Autodesk Inventor part; units mm, degrees
(part 2 of 2)
sketch "Sketch3" plane through (0, 0, 6) normal (0, 0, 1) x (1, 0, 0)
  spline S0 degree 3 poles (20.5297, 43.2466) (22.2295, 43.4705) (23.9405, 43.387) (25.6486, 43.3844) (26.304, 43.3834) (26.9616, 43.2869) (27.6139, 43.2016) (28.7287, 43.056) (29.8441, 42.908) (30.9514, 42.7157) (31.5862, 42.6054) (32.2139, 42.4329) (32.8297, 42.2404) (33.8935, 41.9078) (34.9839, 41.623) (35.9513, 41.0534) (36.6965, 40.6147) (37.4233, 40.1316) (38.101, 39.5959) (38.7184, 39.1078) (39.283, 38.5455) (39.8274, 37.9745) (40.65, 37.1119) (41.2721, 36.1125) (41.7344, 35.009) (41.9858, 34.409) (42.2171, 33.807) (42.3148, 33.1626) (42.3838, 32.7068) (42.4311, 32.2477) (42.4863, 31.7898) (42.5051, 31.6342) (42.5379, 31.4772) (42.5307, 31.3223) (42.5103, 30.883) (42.4889, 30.4426) (42.4376, 30.0063) (42.3757, 29.4795) (42.3242, 28.9459) (42.1926, 28.4346) (42.0204, 27.7655) (41.7834, 27.1124) (41.5557, 26.4588) (41.4533, 26.1649) (41.2846, 25.8939) (41.1845, 25.5995) (41.0297, 25.1443) (40.6487, 24.9481) (40.2751, 24.735) (39.0786, 24.0524) (37.7888, 23.6132) (36.4604, 23.2756) (36.4092, 23.2626) (36.3519, 23.2739) (36.2541, 23.2739) (36.4505, 24.0942) (36.6431, 24.8992) (36.8482, 25.7561) (36.6342, 25.7121) (36.4556, 25.6842) (36.2819, 25.6384) (34.8048, 25.2487) (33.3458, 24.8006) (31.9384, 24.2032) (30.8391, 23.7366) (29.7481, 23.2495) (28.6622, 22.7525) (27.9303, 22.4174) (27.21, 22.0565) (26.4914, 21.6935) (25.9143, 21.4019) (25.3477, 21.0895) (24.7091, 20.7508) (24.8093, 21.0975) (24.9023, 21.38) (24.9722, 21.6681) (25.2788, 22.9311) (25.5986, 24.1916) (25.8741, 25.4615) (26.054, 26.2911) (26.177, 27.1338) (26.3051, 27.9737) (26.3899, 28.5302) (26.4541, 29.091) (26.4995, 29.6521) (26.5622, 30.4281) (26.6152, 31.2056) (26.6412, 31.9834) (26.6645, 32.6834) (26.6815, 33.387) (26.6382, 34.0851) (26.5457, 35.5779) (26.2672, 37.0419) (25.7848, 38.4586) (25.5349, 39.1927) (25.1548, 39.8693) (24.7123, 40.5097) (23.7382, 41.9194) (22.4265, 42.8309) (20.7539, 43.2161) (20.6807, 43.2329) (20.6045, 43.2367) (20.5297, 43.2466) knots 0 0 0 0 1 1 1 2 2 2 3 3 3 4 4 4 5 5 5 6 6 6 7 7 7 8 8 8 9 9 9 10 10 10 11 11 11 12 12 12 13 13 13 14 14 14 15 15 15 16 16 16 17 17 17 18 18 18 19 19 19 20 20 20 21 21 21 22 22 22 23 23 23 24 24 24 25 25 25 26 26 26 27 27 27 28 28 28 29 29 29 30 30 30 31 31 31 32 32 32 33 33 33 34 34 34 34
  line L0 (20.5297, 43.2466) -> (22.2295, 43.4705) construction
  line L1 (22.2295, 43.4705) -> (23.9405, 43.387) construction
  line L2 (23.9405, 43.387) -> (25.6486, 43.3844) construction
  line L3 (25.6486, 43.3844) -> (26.304, 43.3834) construction
  line L4 (26.304, 43.3834) -> (26.9616, 43.2869) construction
  line L5 (26.9616, 43.2869) -> (27.6139, 43.2016) construction
  line L6 (27.6139, 43.2016) -> (28.7287, 43.056) construction
  line L7 (28.7287, 43.056) -> (29.8441, 42.908) construction
  line L8 (29.8441, 42.908) -> (30.9514, 42.7157) construction
  line L9 (30.9514, 42.7157) -> (31.5862, 42.6054) construction
  line L10 (31.5862, 42.6054) -> (32.2139, 42.4329) construction
  line L11 (32.2139, 42.4329) -> (32.8297, 42.2404) construction
  line L12 (32.8297, 42.2404) -> (33.8935, 41.9078) construction
  line L13 (33.8935, 41.9078) -> (34.9839, 41.623) construction
  line L14 (34.9839, 41.623) -> (35.9513, 41.0534) construction
  line L15 (35.9513, 41.0534) -> (36.6965, 40.6147) construction
  line L16 (36.6965, 40.6147) -> (37.4233, 40.1316) construction
  line L17 (37.4233, 40.1316) -> (38.101, 39.5959) construction
  line L18 (38.101, 39.5959) -> (38.7184, 39.1078) construction
  line L19 (38.7184, 39.1078) -> (39.283, 38.5455) construction
  line L20 (39.283, 38.5455) -> (39.8274, 37.9745) construction
  line L21 (39.8274, 37.9745) -> (40.65, 37.1119) construction
  line L22 (40.65, 37.1119) -> (41.2721, 36.1125) construction
  line L23 (41.2721, 36.1125) -> (41.7344, 35.009) construction
  line L24 (41.7344, 35.009) -> (41.9858, 34.409) construction
  line L25 (41.9858, 34.409) -> (42.2171, 33.807) construction
  line L26 (42.2171, 33.807) -> (42.3148, 33.1626) construction
  line L27 (42.3148, 33.1626) -> (42.3838, 32.7068) construction
  line L28 (42.3838, 32.7068) -> (42.4311, 32.2477) construction
  line L29 (42.4311, 32.2477) -> (42.4863, 31.7898) construction
  line L30 (42.4863, 31.7898) -> (42.5051, 31.6342) construction
  line L31 (42.5051, 31.6342) -> (42.5379, 31.4772) construction
  line L32 (42.5379, 31.4772) -> (42.5307, 31.3223) construction
  line L33 (42.5307, 31.3223) -> (42.5103, 30.883) construction
  line L34 (42.5103, 30.883) -> (42.4889, 30.4426) construction
  line L35 (42.4889, 30.4426) -> (42.4376, 30.0063) construction
  line L36 (42.4376, 30.0063) -> (42.3757, 29.4795) construction
  line L37 (42.3757, 29.4795) -> (42.3242, 28.9459) construction
  line L38 (42.3242, 28.9459) -> (42.1926, 28.4346) construction
  line L39 (42.1926, 28.4346) -> (42.0204, 27.7655) construction
  line L40 (42.0204, 27.7655) -> (41.7834, 27.1124) construction
  line L41 (41.7834, 27.1124) -> (41.5557, 26.4588) construction
  line L42 (41.5557, 26.4588) -> (41.4533, 26.1649) construction
  line L43 (41.4533, 26.1649) -> (41.2846, 25.8939) construction
  line L44 (41.2846, 25.8939) -> (41.1845, 25.5995) construction
  line L45 (41.1845, 25.5995) -> (41.0297, 25.1443) construction
  line L46 (41.0297, 25.1443) -> (40.6487, 24.9481) construction
  line L47 (40.6487, 24.9481) -> (40.2751, 24.735) construction
  line L48 (40.2751, 24.735) -> (39.0786, 24.0524) construction
  line L49 (39.0786, 24.0524) -> (37.7888, 23.6132) construction
  line L50 (37.7888, 23.6132) -> (36.4604, 23.2756) construction
  line L51 (36.4604, 23.2756) -> (36.4092, 23.2626) construction
  line L52 (36.4092, 23.2626) -> (36.3519, 23.2739) construction
  line L53 (36.3519, 23.2739) -> (36.2541, 23.2739) construction
  line L54 (36.2541, 23.2739) -> (36.4505, 24.0942) construction
  line L55 (36.4505, 24.0942) -> (36.6431, 24.8992) construction
  line L56 (36.6431, 24.8992) -> (36.8482, 25.7561) construction
  line L57 (36.8482, 25.7561) -> (36.6342, 25.7121) construction
  line L58 (36.6342, 25.7121) -> (36.4556, 25.6842) construction
  line L59 (36.4556, 25.6842) -> (36.2819, 25.6384) construction
  line L60 (36.2819, 25.6384) -> (34.8048, 25.2487) construction
  line L61 (34.8048, 25.2487) -> (33.3458, 24.8006) construction
  line L62 (33.3458, 24.8006) -> (31.9384, 24.2032) construction
  line L63 (31.9384, 24.2032) -> (30.8391, 23.7366) construction
  line L64 (30.8391, 23.7366) -> (29.7481, 23.2495) construction
  line L65 (29.7481, 23.2495) -> (28.6622, 22.7525) construction
  line L66 (28.6622, 22.7525) -> (27.9303, 22.4174) construction
  line L67 (27.9303, 22.4174) -> (27.21, 22.0565) construction
  line L68 (27.21, 22.0565) -> (26.4914, 21.6935) construction
  line L69 (26.4914, 21.6935) -> (25.9143, 21.4019) construction
  line L70 (25.9143, 21.4019) -> (25.3477, 21.0895) construction
  line L71 (25.3477, 21.0895) -> (24.7091, 20.7508) construction
  line L72 (24.7091, 20.7508) -> (24.8093, 21.0975) construction
  line L73 (24.8093, 21.0975) -> (24.9023, 21.38) construction
  line L74 (24.9023, 21.38) -> (24.9722, 21.6681) construction
  line L75 (24.9722, 21.6681) -> (25.2788, 22.9311) construction
  line L76 (25.2788, 22.9311) -> (25.5986, 24.1916) construction
  line L77 (25.5986, 24.1916) -> (25.8741, 25.4615) construction
  line L78 (25.8741, 25.4615) -> (26.054, 26.2911) construction
  line L79 (26.054, 26.2911) -> (26.177, 27.1338) construction
  line L80 (26.177, 27.1338) -> (26.3051, 27.9737) construction
  line L81 (26.3051, 27.9737) -> (26.3899, 28.5302) construction
  line L82 (26.3899, 28.5302) -> (26.4541, 29.091) construction
  line L83 (26.4541, 29.091) -> (26.4995, 29.6521) construction
  line L84 (26.4995, 29.6521) -> (26.5622, 30.4281) construction
  line L85 (26.5622, 30.4281) -> (26.6152, 31.2056) construction
  line L86 (26.6152, 31.2056) -> (26.6412, 31.9834) construction
  line L87 (26.6412, 31.9834) -> (26.6645, 32.6834) construction
  line L88 (26.6645, 32.6834) -> (26.6815, 33.387) construction
  line L89 (26.6815, 33.387) -> (26.6382, 34.0851) construction
  line L90 (26.6382, 34.0851) -> (26.5457, 35.5779) construction
  line L91 (26.5457, 35.5779) -> (26.2672, 37.0419) construction
  line L92 (26.2672, 37.0419) -> (25.7848, 38.4586) construction
  line L93 (25.7848, 38.4586) -> (25.5349, 39.1927) construction
  line L94 (25.5349, 39.1927) -> (25.1548, 39.8693) construction
  line L95 (25.1548, 39.8693) -> (24.7123, 40.5097) construction
  line L96 (24.7123, 40.5097) -> (23.7382, 41.9194) construction
  line L97 (23.7382, 41.9194) -> (22.4265, 42.8309) construction
  line L98 (22.4265, 42.8309) -> (20.7539, 43.2161) construction
  line L99 (20.7539, 43.2161) -> (20.6807, 43.2329) construction
  line L100 (20.6807, 43.2329) -> (20.6045, 43.2367) construction
  line L101 (20.6045, 43.2367) -> (20.5297, 43.2466) construction
  spline S1 degree 3 poles (36.6036, 23.5895) (37.0569, 23.702) (37.5183, 23.7768) (37.9504, 23.9327) (38.6597, 24.1886) (39.3668, 24.4661) (39.9357, 24.9927) (40.1802, 25.219) (40.2083, 25.5928) (39.8107, 25.7537) (39.4496, 25.8997) (39.0786, 25.933) (38.6918, 25.8914) (38.254, 25.8443) (37.8103, 25.844) (37.3764, 25.7764) (37.2463, 25.7562) (37.07, 25.5981) (37.0357, 25.4707) (36.8712, 24.8601) (36.7483, 24.2385) (36.6036, 23.5895) knots 0 0 0 0 1 1 1 2 2 2 3 3 3 4 4 4 5 5 5 6 6 6 7 7 7 7
  line L102 (36.6036, 23.5895) -> (37.0569, 23.702) construction
  line L103 (37.0569, 23.702) -> (37.5183, 23.7768) construction
  line L104 (37.5183, 23.7768) -> (37.9504, 23.9327) construction
  line L105 (37.9504, 23.9327) -> (38.6597, 24.1886) construction
  line L106 (38.6597, 24.1886) -> (39.3668, 24.4661) construction
  line L107 (39.3668, 24.4661) -> (39.9357, 24.9927) construction
  line L108 (39.9357, 24.9927) -> (40.1802, 25.219) construction
  line L109 (40.1802, 25.219) -> (40.2083, 25.5928) construction
  line L110 (40.2083, 25.5928) -> (39.8107, 25.7537) construction
  line L111 (39.8107, 25.7537) -> (39.4496, 25.8997) construction
  line L112 (39.4496, 25.8997) -> (39.0786, 25.933) construction
  line L113 (39.0786, 25.933) -> (38.6918, 25.8914) construction
  line L114 (38.6918, 25.8914) -> (38.254, 25.8443) construction
  line L115 (38.254, 25.8443) -> (37.8103, 25.844) construction
  line L116 (37.8103, 25.844) -> (37.3764, 25.7764) construction
  line L117 (37.3764, 25.7764) -> (37.2463, 25.7562) construction
  line L118 (37.2463, 25.7562) -> (37.07, 25.5981) construction
  line L119 (37.07, 25.5981) -> (37.0357, 25.4707) construction
  line L120 (37.0357, 25.4707) -> (36.8712, 24.8601) construction
  line L121 (36.8712, 24.8601) -> (36.7483, 24.2385) construction
  line L122 (36.7483, 24.2385) -> (36.6036, 23.5895) construction
  line L123 (20.3717, 33.3225) -> (30.5343, 33.3225) construction
  line L124 (30.5343, 33.3225) -> (30.5343, 28.6993) construction
  line L125 (30.5343, 28.6993) -> (20.3717, 28.6993) construction
  line L126 (20.3717, 28.6993) -> (20.3717, 33.3225) construction
  spline S2 degree 2 poles (21.5765, 30.0395) (21.2323, 30.0395) (20.7494, 30.1833) (20.5361, 30.2861) knots 0 0 0 1 2 2 2
  line L127 (20.5361, 30.2861) -> (20.5361, 30.8153)
  line L128 (20.5361, 30.8153) -> (20.567, 30.8153)
  spline S3 degree 2 poles (20.567, 30.8153) (20.7751, 30.62) (21.3017, 30.4043) (21.5457, 30.4043) knots 0 0 0 1 2 2 2
  spline S4 degree 2 poles (21.5457, 30.4043) (21.8951, 30.4043) (22.2522, 30.6945) (22.2522, 30.9334) knots 0 0 0 1 2 2 2
  spline S5 degree 2 poles (22.2522, 30.9334) (22.2522, 31.1235) (22.0646, 31.3599) (21.8617, 31.419) knots 0 0 0 1 2 2 2
  spline S6 degree 2 poles (21.8617, 31.419) (21.7153, 31.4601) (21.4712, 31.5166) (21.2888, 31.5628) knots 0 0 0 1 2 2 2
  spline S7 degree 2 poles (21.2888, 31.5628) (21.1244, 31.6065) (20.865, 31.7375) (20.7648, 31.8428) knots 0 0 0 1 2 2 2
  spline S8 degree 2 poles (20.7648, 31.8428) (20.6672, 31.9482) (20.5593, 32.2307) (20.5593, 32.4157) knots 0 0 0 1 2 2 2
  spline S9 degree 2 poles (20.5593, 32.4157) (20.5593, 32.801) (21.1604, 33.3225) (21.6254, 33.3225) knots 0 0 0 1 2 2 2
  spline S10 degree 2 poles (21.6254, 33.3225) (21.8925, 33.3225) (22.3652, 33.2172) (22.5681, 33.117) knots 0 0 0 1 2 2 2
  line L129 (22.5681, 33.117) -> (22.5681, 32.6135)
  line L130 (22.5681, 32.6135) -> (22.5373, 32.6135)
  spline S11 degree 2 poles (22.5373, 32.6135) (22.3857, 32.7522) (21.9131, 32.9577) (21.6536, 32.9577) knots 0 0 0 1 2 2 2
  spline S12 degree 2 poles (21.6536, 32.9577) (21.3608, 32.9577) (20.9985, 32.6829) (20.9985, 32.4594) knots 0 0 0 1 2 2 2
  spline S13 degree 2 poles (20.9985, 32.4594) (20.9985, 32.259) (21.2118, 32.0201) (21.4121, 31.9661) knots 0 0 0 1 2 2 2
  spline S14 degree 2 poles (21.4121, 31.9661) (21.5457, 31.9302) (21.9336, 31.8377) (22.0621, 31.7992) knots 0 0 0 1 2 2 2
  spline S15 degree 2 poles (22.0621, 31.7992) (22.3883, 31.699) (22.6914, 31.2957) (22.6914, 31.0002) knots 0 0 0 1 2 2 2
  spline S16 degree 2 poles (22.6914, 31.0002) (22.6914, 30.8127) (22.5399, 30.4531) (22.4037, 30.3272) knots 0 0 0 1 2 2 2
  spline S17 degree 2 poles (22.4037, 30.3272) (22.2522, 30.1885) (21.8668, 30.0395) (21.5765, 30.0395) knots 0 0 0 1 2 2 2
  spline S18 degree 2 poles (25.0831, 31.3496) (25.0831, 30.7536) (24.5153, 30.0497) (24.0812, 30.0497) knots 0 0 0 1 2 2 2
  spline S19 degree 2 poles (24.0812, 30.0497) (23.904, 30.0497) (23.6316, 30.132) (23.4904, 30.2167) knots 0 0 0 1 2 2 2
  line L131 (23.4904, 30.2167) -> (23.4904, 29.22)
  line L132 (23.4904, 29.22) -> (23.0896, 29.22)
  line L133 (23.0896, 29.22) -> (23.0896, 32.4748)
  line L134 (23.0896, 32.4748) -> (23.4904, 32.4748)
  line L135 (23.4904, 32.4748) -> (23.4904, 32.2256)
  spline S20 degree 2 poles (23.4904, 32.2256) (23.6394, 32.3617) (24.0041, 32.5416) (24.2174, 32.5416) knots 0 0 0 1 2 2 2
  spline S21 degree 2 poles (24.2174, 32.5416) (24.6258, 32.5416) (25.0831, 31.8942) (25.0831, 31.3496) knots 0 0 0 1 2 2 2
  spline S22 degree 2 poles (24.6695, 31.3034) (24.6695, 31.7118) (24.41, 32.1614) (24.1197, 32.1614) knots 0 0 0 1 2 2 2
  spline S23 degree 2 poles (24.1197, 32.1614) (23.9502, 32.1614) (23.6316, 32.0098) (23.4904, 31.8916) knots 0 0 0 1 2 2 2
  line L136 (23.4904, 31.8916) -> (23.4904, 30.5404)
  spline S24 degree 2 poles (23.4904, 30.5404) (23.6471, 30.4659) (23.8706, 30.4094) (24.0144, 30.4094) knots 0 0 0 1 2 2 2
  spline S25 degree 2 poles (24.0144, 30.4094) (24.3252, 30.4094) (24.6695, 30.8667) (24.6695, 31.3034) knots 0 0 0 1 2 2 2
  line L137 (25.9077, 30.096) -> (25.5069, 30.096)
  line L138 (25.5069, 30.096) -> (25.5069, 32.4748)
  line L139 (25.5069, 32.4748) -> (25.9077, 32.4748)
  line L140 (25.9077, 32.4748) -> (25.9077, 30.096)
  line L141 (25.9359, 32.8704) -> (25.4812, 32.8704)
  line L142 (25.4812, 32.8704) -> (25.4812, 33.2865)
  line L143 (25.4812, 33.2865) -> (25.9359, 33.2865)
  line L144 (25.9359, 33.2865) -> (25.9359, 32.8704)
  point P0 (-33.7147, -35.2257)
  point P1 (-33.0448, -40.4532)
  point P2 (-33.7217, -38.9912)
  point P3 (-33.1276, -39.7943)
  point P4 (-39.3868, -42.9109)
  point P5 (0, 0)
  constraints: 5 other
extrude "Extrusion4" cut sketch "Sketch3" against normal blind 0.5
sketch "Sketch4" plane through (0, 0, 6) normal (0, 0, 1) x (1, 0, 0)
  line L0 (26.9346, 33.3438) -> (41.0814, 33.3438) construction
  line L1 (41.0814, 33.3438) -> (41.0814, 29.9657) construction
  line L2 (41.0814, 29.9657) -> (26.9346, 29.9657) construction
  line L3 (26.9346, 29.9657) -> (26.9346, 33.3438) construction
  line L4 (29.524, 30.0325) -> (29.0513, 30.0325)
  line L5 (29.0513, 30.0325) -> (27.6487, 32.7658)
  line L6 (27.6487, 32.7658) -> (27.6487, 30.0325)
  line L7 (27.6487, 30.0325) -> (27.2557, 30.0325)
  line L8 (27.2557, 30.0325) -> (27.2557, 33.2025)
  line L9 (27.2557, 33.2025) -> (27.8542, 33.2025)
  line L10 (27.8542, 33.2025) -> (29.131, 30.6927)
  line L11 (29.131, 30.6927) -> (29.131, 33.2025)
  line L12 (29.131, 33.2025) -> (29.524, 33.2025)
  line L13 (29.524, 33.2025) -> (29.524, 30.0325)
  line L14 (32.4346, 30.0325) -> (31.9619, 30.0325)
  line L15 (31.9619, 30.0325) -> (30.5593, 32.7658)
  line L16 (30.5593, 32.7658) -> (30.5593, 30.0325)
  line L17 (30.5593, 30.0325) -> (30.1662, 30.0325)
  line L18 (30.1662, 30.0325) -> (30.1662, 33.2025)
  line L19 (30.1662, 33.2025) -> (30.7648, 33.2025)
  line L20 (30.7648, 33.2025) -> (32.0415, 30.6927)
  line L21 (32.0415, 30.6927) -> (32.0415, 33.2025)
  line L22 (32.0415, 33.2025) -> (32.4346, 33.2025)
  line L23 (32.4346, 33.2025) -> (32.4346, 30.0325)
  spline S0 degree 2 poles (34.3715, 30.2843) (34.3227, 30.2483) (34.1583, 30.1199) (34.0812, 30.0813) knots 0 0 0 1 2 2 2
  spline S1 degree 2 poles (34.0812, 30.0813) (33.9759, 30.0248) (33.7781, 29.9657) (33.5983, 29.9657) knots 0 0 0 1 2 2 2
  spline S2 degree 2 poles (33.5983, 29.9657) (33.4518, 29.9657) (33.1872, 30.0762) (33.0871, 30.1764) knots 0 0 0 1 2 2 2
  spline S3 degree 2 poles (33.0871, 30.1764) (32.992, 30.274) (32.8764, 30.5617) (32.8764, 30.721) knots 0 0 0 1 2 2 2
  spline S4 degree 2 poles (32.8764, 30.721) (32.8764, 30.9676) (33.0845, 31.317) (33.3105, 31.4171) knots 0 0 0 1 2 2 2
  spline S5 degree 2 poles (33.3105, 31.4171) (33.5109, 31.5096) (34.0555, 31.579) (34.3715, 31.597) knots 0 0 0 1 2 2 2
  line L24 (34.3715, 31.597) -> (34.3715, 31.674)
  spline S6 degree 2 poles (34.3715, 31.674) (34.3715, 31.8128) (34.2867, 31.9849) (34.2097, 32.0337) knots 0 0 0 1 2 2 2
  spline S7 degree 2 poles (34.2097, 32.0337) (34.1326, 32.0825) (33.9117, 32.1133) (33.7935, 32.1133) knots 0 0 0 1 2 2 2
  spline S8 degree 2 poles (33.7935, 32.1133) (33.6548, 32.1133) (33.2797, 32.0311) (33.0922, 31.9515) knots 0 0 0 1 2 2 2
  line L25 (33.0922, 31.9515) -> (33.0691, 31.9515)
  line L26 (33.0691, 31.9515) -> (33.0691, 32.3599)
  spline S9 degree 2 poles (33.0691, 32.3599) (33.1795, 32.3908) (33.5931, 32.4678) (33.7961, 32.4678) knots 0 0 0 1 2 2 2
  spline S10 degree 2 poles (33.7961, 32.4678) (34.0427, 32.4678) (34.3792, 32.3908) (34.5128, 32.2906) knots 0 0 0 1 2 2 2
  spline S11 degree 2 poles (34.5128, 32.2906) (34.6438, 32.193) (34.7722, 31.8821) (34.7722, 31.6586) knots 0 0 0 1 2 2 2
  line L27 (34.7722, 31.6586) -> (34.7722, 30.0325)
  line L28 (34.7722, 30.0325) -> (34.3715, 30.0325)
  line L29 (34.3715, 30.0325) -> (34.3715, 30.2843)
  line L30 (34.3715, 30.6182) -> (34.3715, 31.2784)
  spline S12 degree 2 poles (34.3715, 31.2784) (34.2276, 31.2656) (33.7935, 31.2219) (33.6573, 31.1808) knots 0 0 0 1 2 2 2
  spline S13 degree 2 poles (33.6573, 31.1808) (33.4981, 31.132) (33.29, 30.9291) (33.29, 30.7492) knots 0 0 0 1 2 2 2
  spline S14 degree 2 poles (33.29, 30.7492) (33.29, 30.5437) (33.5212, 30.3357) (33.7421, 30.3357) knots 0 0 0 1 2 2 2
  spline S15 degree 2 poles (33.7421, 30.3357) (33.9296, 30.3357) (34.2379, 30.4975) (34.3715, 30.6182) knots 0 0 0 1 2 2 2
  line L31 (37.3052, 30.0325) -> (36.7785, 30.0325)
  line L32 (36.7785, 30.0325) -> (35.8948, 31.1808)
  line L33 (35.8948, 31.1808) -> (35.7356, 31.0267)
  line L34 (35.7356, 31.0267) -> (35.7356, 30.0325)
  line L35 (35.7356, 30.0325) -> (35.3348, 30.0325)
  line L36 (35.3348, 30.0325) -> (35.3348, 33.3438)
  line L37 (35.3348, 33.3438) -> (35.7356, 33.3438)
  line L38 (35.7356, 33.3438) -> (35.7356, 31.4069)
  line L39 (35.7356, 31.4069) -> (36.6758, 32.4113)
  line L40 (36.6758, 32.4113) -> (37.1741, 32.4113)
  line L41 (37.1741, 32.4113) -> (36.198, 31.4171)
  line L42 (36.198, 31.4171) -> (37.3052, 30.0325)
  spline S16 degree 2 poles (38.5382, 29.9786) (37.9679, 29.9786) (37.3411, 30.6182) (37.3411, 31.2091) knots 0 0 0 1 2 2 2
  spline S17 degree 2 poles (37.3411, 31.2091) (37.3411, 31.7896) (37.9499, 32.4781) (38.4406, 32.4781) knots 0 0 0 1 2 2 2
  spline S18 degree 2 poles (38.4406, 32.4781) (38.6615, 32.4781) (39.0032, 32.3497) (39.1291, 32.2135) knots 0 0 0 1 2 2 2
  spline S19 degree 2 poles (39.1291, 32.2135) (39.2575, 32.0774) (39.3937, 31.6843) (39.3937, 31.3992) knots 0 0 0 1 2 2 2
  line L43 (39.3937, 31.3992) -> (39.3937, 31.1808)
  line L44 (39.3937, 31.1808) -> (37.747, 31.1808)
  spline S20 degree 2 poles (37.747, 31.1808) (37.747, 30.7672) (38.1632, 30.3279) (38.5331, 30.3279) knots 0 0 0 1 2 2 2
  spline S21 degree 2 poles (38.5331, 30.3279) (38.6641, 30.3279) (38.9184, 30.387) (39.0212, 30.4333) knots 0 0 0 1 2 2 2
  spline S22 degree 2 poles (39.0212, 30.4333) (39.1291, 30.4846) (39.2781, 30.5746) (39.3269, 30.6157) knots 0 0 0 1 2 2 2
  line L45 (39.3269, 30.6157) -> (39.35, 30.6157)
  line L46 (39.35, 30.6157) -> (39.35, 30.1789)
  spline S23 degree 2 poles (39.35, 30.1789) (39.2806, 30.1507) (39.07, 30.0685) (38.9878, 30.0454) knots 0 0 0 1 2 2 2
  spline S24 degree 2 poles (38.9878, 30.0454) (38.8722, 30.012) (38.6821, 29.9786) (38.5382, 29.9786) knots 0 0 0 1 2 2 2
  spline S25 degree 2 poles (39.0032, 31.4865) (38.9981, 31.6483) (38.9313, 31.8847) (38.867, 31.9643) knots 0 0 0 1 2 2 2
  spline S26 degree 2 poles (38.867, 31.9643) (38.7977, 32.0542) (38.5793, 32.1493) (38.4175, 32.1493) knots 0 0 0 1 2 2 2
  spline S27 degree 2 poles (38.4175, 32.1493) (38.2582, 32.1493) (38.0347, 32.0542) (37.9422, 31.9618) knots 0 0 0 1 2 2 2
  spline S28 degree 2 poles (37.9422, 31.9618) (37.8523, 31.8667) (37.7599, 31.6381) (37.747, 31.4865) knots 0 0 0 1 2 2 2
  line L47 (37.747, 31.4865) -> (39.0032, 31.4865)
  line L48 (41.0609, 31.9823) -> (41.0403, 31.9823)
  spline S29 degree 2 poles (41.0403, 31.9823) (40.9941, 31.9951) (40.8939, 32.0003) (40.8245, 32.0003) knots 0 0 0 1 2 2 2
  spline S30 degree 2 poles (40.8245, 32.0003) (40.6627, 32.0003) (40.3441, 31.859) (40.2003, 31.7203) knots 0 0 0 1 2 2 2
  line L49 (40.2003, 31.7203) -> (40.2003, 30.0325)
  line L50 (40.2003, 30.0325) -> (39.7995, 30.0325)
  line L51 (39.7995, 30.0325) -> (39.7995, 32.4113)
  line L52 (39.7995, 32.4113) -> (40.2003, 32.4113)
  line L53 (40.2003, 32.4113) -> (40.2003, 32.0568)
  spline S31 degree 2 poles (40.2003, 32.0568) (40.4186, 32.252) (40.7449, 32.4113) (40.899, 32.4113) knots 0 0 0 1 2 2 2
  spline S32 degree 2 poles (40.899, 32.4113) (40.9607, 32.4113) (41.0223, 32.4062) (41.0609, 32.3985) knots 0 0 0 1 2 2 2
  line L54 (41.0609, 32.3985) -> (41.0609, 31.9823)
  point P0 (-33.7147, -35.2257)
  point P1 (-33.0448, -40.4532)
  point P2 (-33.7217, -38.9912)
  point P3 (-33.1276, -39.7943)
  point P4 (-39.3868, -42.9109)
  point P5 (0, 0)
  constraints: 2 other
extrude "Extrusion5" add sketch "Sketch4" along normal blind 0.5
body "Solid1"
